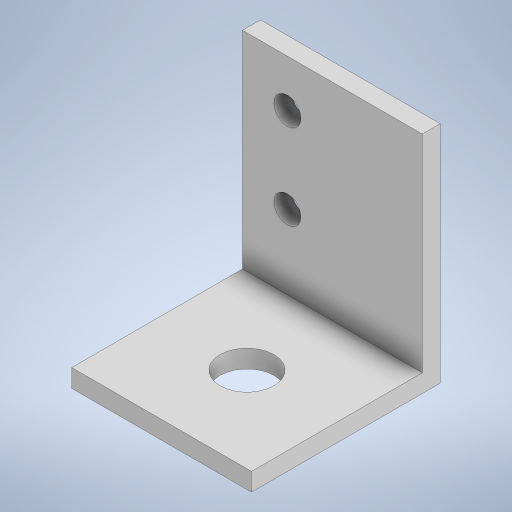
# Autodesk Inventor part: LimitSwitch Mount
Saved by Autodesk Inventor 2023 (Build 270158000, 158)
## iProperties
Created: 2023-04-27
Part Number: LimitSwitch Mount
Material: Generic
Document SubType Name: Modeling
Designer: ethan
Density: 1 g/cm^3
Appearance: Default
Author: ethan
Autodesk Inventor part; units mm, degrees
ref_plane "YZ Plane" through (0, 0, 0) normal (1, 0, 0) x (0, 1, 0)
ref_plane "XZ Plane" through (0, 0, 0) normal (0, 1, 0) x (-1, 0, 0)
ref_plane "XY Plane" through (0, 0, 0) normal (0, 0, 1) x (1, 0, 0)
sketch "Sketch1" plane through (0, 0, 0) normal (0, 0, 1) x (1, 0, 0)
  line L0 (0, 0) -> (-20, 0)
  line L1 (-20, 0) -> (-20, 25)
  line L2 (-20, 25) -> (0, 25)
  line L3 (0, 25) -> (0, 0)
  circle A0 centre (-15, 19.75) radius 1.5
  circle A1 centre (-15, 10.25) radius 1.5
  dimension "d0" = 20
  dimension "d1" = 25
  dimension "d7" = 3
  dimension "d8" = 3
  dimension "d9" = 9.5
  dimension "d10" = 15
  dimension "d11" = 5.25
  constraints: 8 end point, 2 centre point, 2 parallel, 1 horizontal, 1 perpendicular
  measures "d0" distance of L1.end L2.end
  measures "d1" distance of L0.end L1.end
  measures "d7" diameter of A0
  measures "d8" diameter of A1
  measures "d9" distance of A1.centre A0.centre
  measures "d10" distance from line of L3 A0.centre
  measures "d11" distance from line of L2 A0.centre
extrude "Extrusion1" add sketch "Sketch1" along normal blind 2
sketch "Sketch2" plane through (0, 0, 2) normal (0, 0, 1) x (1, 0, 0)
  line L0 (-20, 25) -> (-20, 0) projected
  line L1 (0, 0) -> (0, 25) projected
  line L2 (-20, 0) -> (0, 0)
  line L3 (0, 0) -> (0, 2)
  line L4 (0, 2) -> (-20, 2)
  line L5 (-20, 2) -> (-20, 0)
  dimension "d4" = 2
  constraints: 8 end point, 2 parallel, 1 horizontal, 1 perpendicular, 1 point on line
  measures "d4" distance of L3.end L2.end
extrude "Extrusion2" add sketch "Sketch2" along normal blind 19
sketch "Sketch3" plane through (-20, 2, 2) normal (0, 1, 0) x (1, 0, 0)
  line L0 (0, -19) -> (20, -19) construction
  line L1 (20, -19) -> (0, 0) construction
  circle A0 centre (10, -9.5) radius 3
  point P0 (20, 2)
  dimension "d12" = 6
  constraints: 2 end point, 1 centre point, 1 midpoint
  measures "d12" diameter of A0
extrude "Extrusion3" cut sketch "Sketch3" against normal blind 2
body "Solid1"
